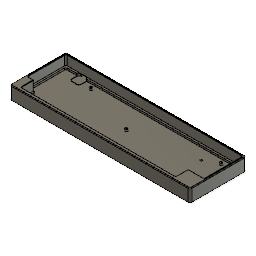
ttocyobitna (Autodesk Fusion 360 design; units mm, degrees)
Autodesk Fusion 360 part; units mm, degrees
sketch "Sketch1" plane through (0, 0, 0) normal (0, 1, 0) x (1, 0, 0)
  line L0 (0, 0) -> (274.2, 0)
  line L1 (274.2, 0) -> (274.2, -85.7)
  line L2 (274.2, -85.7) -> (0, -85.7)
  line L3 (0, -85.7) -> (0, 0)
  dimension "d1" = 274.2
  dimension "d2" = 85.7
  constraint horizontal L0
  constraint vertical L1
  constraint horizontal L2
  constraint vertical L3
  constraint coincident L0.start L3.end
  measures "d1" distance of L0.start L0.end
  measures "d2" distance of L0.start L2.end
extrude "Extrude1" add sketch "Sketch1" along normal blind 20.5
sketch "Sketch2" plane through (0, 20.5, 0) normal (0, 1, 0) x (-1, 0, 0)
  line L0 (0, 85.7) -> (-274.2, 85.7)
  line L1 (-274.2, 85.7) -> (-274.2, 0)
  line L2 (-274.2, 0) -> (0, 0)
  line L3 (0, 0) -> (0, 85.7)
  line L4 (-5, 3) -> (-269.2, 3)
  line L5 (-271.2, 5) -> (-271.2, 78.7)
  line L6 (-269.2, 80.7) -> (-5, 80.7)
  line L7 (-3, 78.7) -> (-3, 5)
  arc A0 (-5, 3) -> (-3, 5) centre (-5, 5) ccw
  arc A1 (-3, 78.7) -> (-5, 80.7) centre (-5, 78.7) ccw
  arc A2 (-269.2, 80.7) -> (-271.2, 78.7) centre (-269.2, 78.7) ccw
  arc A3 (-271.2, 5) -> (-269.2, 3) centre (-269.2, 5) ccw
  dimension "d5" = 3
  dimension "d6" = 5
  dimension "d7" = 3
  dimension "d8" = 3
  dimension "d9" = 2
  constraint horizontal L4
  constraint vertical L5
  constraint horizontal L6
  constraint vertical L7
  constraint tangent L4 A0
  constraint tangent L7 A0
  constraint tangent L6 A1
  constraint tangent L7 A1
  constraint equal A0 A1
  constraint tangent L5 A2
  constraint tangent L6 A2
  constraint equal A0 A2
  constraint tangent L4 A3
  constraint tangent L5 A3
  constraint equal A0 A3
  measures "d5" distance of L1 L5
  measures "d6" distance of L0 L6
  measures "d7" distance of L2 L4
  measures "d8" distance of L3 L7
  measures "d9" radius of A0
extrude "Extrude2" cut sketch "Sketch2" against normal blind 17.23 contours L4 L5 L6 L7 A0 A1 A2 A3
sketch "Sketch3" plane through (0, 3.27, 0) normal (0, 1, 0) x (-1, 0, 0)
  arc A0 (-269.2, 80.7) -> (-271.2, 78.7) centre (-269.2, 78.7) ccw
  line L0 (-271.2, 78.7) -> (-271.2, 5)
  arc A1 (-271.2, 5) -> (-269.2, 3) centre (-269.2, 5) ccw
  line L1 (-269.2, 3) -> (-5, 3)
  arc A2 (-5, 3) -> (-3, 5) centre (-5, 5) ccw
  line L2 (-3, 5) -> (-3, 78.7)
  arc A3 (-3, 78.7) -> (-5, 80.7) centre (-5, 78.7) ccw
  line L3 (-5, 80.7) -> (-269.2, 80.7)
  circle A4 centre (-51.375, 13.275) radius 2
  circle A5 centre (-36.275, 70.425) radius 2
  circle A6 centre (-132.3375, 40.775) radius 2
  circle A7 centre (-223.775, 70.425) radius 2
  circle A8 centre (-249.0188, 13.275) radius 2
  circle A9 centre (-228.275, 22.8) radius 1.5875
  line L4 (-7.75, 5.75) -> (-266.45, 5.75)
  line L5 (-268.45, 7.75) -> (-268.45, 75.95)
  line L6 (-266.45, 77.95) -> (-7.75, 77.95)
  line L7 (-5.75, 75.95) -> (-5.75, 7.75)
  arc A10 (-7.75, 5.75) -> (-5.75, 7.75) centre (-7.75, 7.75) ccw
  arc A11 (-5.75, 75.95) -> (-7.75, 77.95) centre (-7.75, 75.95) ccw
  arc A12 (-268.45, 7.75) -> (-266.45, 5.75) centre (-266.45, 7.75) ccw
  arc A13 (-266.45, 77.95) -> (-268.45, 75.95) centre (-266.45, 75.95) ccw
  line L8 (-22.9438, 3) -> (-36.9438, 3)
  line L9 (-36.9438, 3) -> (-36.9438, 17)
  line L10 (-36.9438, 17) -> (-22.9438, 17)
  line L11 (-22.9438, 17) -> (-22.9438, 3)
  point P0 (-13.275, 13.275)
  point P1 (-29.9438, 13.275)
  dimension "d12" = 10.275
  dimension "d13" = 10.275
  dimension "d14" = 4
  dimension "d15" = 38.1
  dimension "d16" = 4
  dimension "d17" = 57.15
  dimension "d18" = 23
  dimension "d19" = 4
  dimension "d20" = 4
  dimension "d21" = 4
  dimension "d22" = 119.0625
  dimension "d23" = 27.5
  dimension "d24" = 235.7438
  dimension "d25" = 210.5
  dimension "d26" = 57.15
  dimension "d27" = 3.175
  dimension "d28" = 215
  dimension "d29" = 9.525
  dimension "d30" = 2.75
  dimension "d31" = 2.75
  dimension "d32" = 2.75
  dimension "d33" = 2.75
  dimension "d34" = 2
  dimension "d41" = 16.6687
  dimension "d43" = 14
  dimension "d44" = 14
  dimension "d45" = 7
  constraint horizontal L4
  constraint vertical L5
  constraint horizontal L6
  constraint vertical L7
  constraint tangent L4 A10
  constraint tangent L7 A10
  constraint tangent L6 A11
  constraint tangent L7 A11
  constraint equal A10 A11
  constraint tangent L4 A12
  constraint tangent L5 A12
  constraint equal A10 A12
  constraint tangent L5 A13
  constraint tangent L6 A13
  constraint equal A10 A13
  constraint horizontal L8
  constraint vertical L9
  constraint horizontal L10
  constraint vertical L11
  constraint coincident L1 L8.start
  measures "d12" distance of L1 P0
  measures "d13" distance of L2 P0
  measures "d14" diameter of A4
  measures "d15" distance of P0 A4.centre
  measures "d16" diameter of A5
  measures "d17" vertical distance of P0 A5.centre
  measures "d18" horizontal distance of P0 A5.centre
  measures "d19" diameter of A6
  measures "d20" diameter of A7
  measures "d21" diameter of A8
  measures "d22" horizontal distance of P0 A6.centre
  measures "d23" vertical distance of P0 A6.centre
  measures "d24" distance of P0 A8.centre
  measures "d25" horizontal distance of P0 A7.centre
  measures "d26" vertical distance of P0 A7.centre
  measures "d27" diameter of A9
  measures "d28" horizontal distance of P0 A9.centre
  measures "d29" vertical distance of P0 A9.centre
  measures "d30" distance of L1 L4
  measures "d31" distance of L0 L5
  measures "d32" distance of L3 L6
  measures "d33" distance of L2 L7
  measures "d34" radius of A10
  measures "d41" distance of P0 P1
  measures "d43" distance of L8.start L8.end
  measures "d44" distance of L8.start L10.end
  measures "d45" distance of P1 L11
extrude "Extrude5" cut sketch "Sketch3" against normal blind 0.52 contours L1 L4 L8 L9 L11 | L4 L9 L10 L11
extrude "Extrude3" add sketch "Sketch3" along normal blind 2.73 contours A0 L0 A1 L1 A2 L2 A3 L3 L4 L5 L6 L7 A10 A11 A12 A13 L9 L11 | L1 L4 L8 L9 L11 | A4 | A5 | A6 | A7 | A8
extrude "Extrude4" cut sketch "Sketch3" against normal blind 3.27 contours A9
sketch "Sketch4" plane through (0, 0, 0) normal (0, 0, -1) x (-1, 0, 0)
  line L0 (-274.2, 0) -> (0, 0)
  line L1 (0, 0) -> (0, 20.5)
  line L2 (0, 20.5) -> (-274.2, 20.5)
  line L3 (-274.2, 20.5) -> (-274.2, 0)
  line L4 (-33.4438, 6.25) -> (-26.4438, 6.25)
  line L5 (-25.4438, 5.25) -> (-25.4438, 3.75)
  line L6 (-26.4438, 2.75) -> (-33.4437, 2.75)
  line L7 (-34.4438, 3.75) -> (-34.4437, 5.25)
  arc A0 (-33.4438, 6.25) -> (-34.4438, 5.25) centre (-33.4438, 5.25) ccw
  arc A1 (-34.4438, 3.75) -> (-33.4438, 2.75) centre (-33.4438, 3.75) ccw
  arc A2 (-26.4438, 2.75) -> (-25.4438, 3.75) centre (-26.4438, 3.75) ccw
  arc A3 (-25.4438, 5.25) -> (-26.4438, 6.25) centre (-26.4438, 5.25) ccw
  point P0 (-55.875, 6.25)
  point P1 (-55.875, 2.75)
  point P2 (-51.375, 3.27)
  point P3 (-34.4438, 6.25)
  point P4 (-25.4438, 6.25)
  point P5 (-34.4438, 2.75)
  point P6 (-29.9438, 3.27)
  dimension "d53" = 9
  dimension "d54" = 3.5
  dimension "d55" = 4.5
  dimension "d56" = 2.98
  dimension "d57" = 1
  constraint horizontal L4
  constraint vertical L5
  constraint horizontal L6
  constraint vertical L7
  constraint coincident P3 L4
  constraint coincident P3 L7
  constraint tangent L4 A0
  constraint tangent L7 A0
  constraint coincident P5 L6
  constraint coincident P5 L7
  constraint tangent L6 A1
  constraint tangent L7 A1
  constraint equal A0 A1
  constraint tangent L5 A2
  constraint tangent L6 A2
  constraint equal A0 A2
  constraint coincident P4 L4
  constraint coincident P4 L5
  constraint tangent L4 A3
  constraint tangent L5 A3
  constraint equal A0 A3
  measures "d53" distance of P3 P4
  measures "d54" distance of P3 P5
  measures "d55" distance of L5 P6
  measures "d56" distance of L4 P6
  measures "d57" radius of A0
extrude "Extrude6" cut sketch "Sketch4" against normal blind 3 contours L4 L5 L6 L7 A0 A1 A2 A3
extrude "Extrude7" cut sketch "Sketch3" along normal blind 2.73 contours L1 L4 L8 L9 L11
fillet "Fillet1" radius 3.175 1 edges at (22.9438, 4.375, 3)
fillet "Fillet2" radius 3.175 1 edges at (36.9438, 4.375, 3)
fillet "Fillet3" radius 3.175 2 edges at (36.9438, 3.01, 17) (22.9438, 3.01, 17)
sketch "Sketch5" plane through (0, 20.5, 0) normal (0, 1, 0) x (-1, 0, 0)
  line L0 (-271.2, 5) -> (-271.2, 78.7)
  arc A0 (-269.2, 80.7) -> (-271.2, 78.7) centre (-269.2, 78.7) ccw
  line L1 (-269.2, 80.7) -> (-5, 80.7)
  arc A1 (-3, 78.7) -> (-5, 80.7) centre (-5, 78.7) ccw
  line L2 (-3, 78.7) -> (-3, 5)
  arc A2 (-5, 3) -> (-3, 5) centre (-5, 5) ccw
  line L3 (-5, 3) -> (-269.2, 3)
  arc A3 (-271.2, 5) -> (-269.2, 3) centre (-269.2, 5) ccw
  line L4 (0, 85.7) -> (-274.2, 85.7)
  line L5 (-274.2, 85.7) -> (-274.2, 0)
  line L6 (-274.2, 0) -> (0, 0)
  line L7 (0, 0) -> (0, 85.7)
  line L8 (-12.525, 80.7) -> (-3, 80.7)
  line L9 (-3, 80.7) -> (-3, 61.65)
  line L10 (-3, 61.65) -> (-12.525, 61.65)
  line L11 (-12.525, 61.65) -> (-12.525, 80.7)
  line L12 (-271.2, 61.65) -> (-247.3875, 61.65)
  line L13 (-247.3875, 61.65) -> (-247.3875, 80.7)
  line L14 (-247.3875, 80.7) -> (-271.2, 80.7)
  line L15 (-271.2, 80.7) -> (-271.2, 61.65)
  dimension "d65" = 9.525
  dimension "d66" = 19.05
  dimension "d67" = 19.05
  dimension "d68" = 23.8125
  constraint horizontal L8
  constraint vertical L9
  constraint horizontal L10
  constraint vertical L11
  constraint coincident L2 L9.end
  constraint horizontal L12
  constraint vertical L13
  constraint horizontal L14
  constraint vertical L15
  constraint coincident L1 L13.end
  constraint coincident L0 L12.start
  measures "d65" distance of L9.end L10.end
  measures "d66" distance of L8.start L10.end
  measures "d67" distance of L12.end L13.end
  measures "d68" distance of L12.start L12.end
extrude "Extrude8" add sketch "Sketch5" against normal blind 20.5 contours L0 A0 L1 L12 L13 L14 L15 | L1 A1 L2 L8 L9 L10 L11
fillet "Fillet4" radius 2 2 edges at (3, 13.25, 61.65) (12.525, 13.25, 80.7)
fillet "Fillet5" radius 2 2 edges at (271.2, 13.25, 61.65) (247.3875, 13.25, 80.7)
fillet "Fillet6" radius 0.5 1 edges at (247.3875, 11.885, 61.65)
fillet "Fillet7" radius 0.5 1 edges at (12.525, 11.885, 61.65)
sketch "Sketch6" plane through (0, 3.27, 0) normal (0, 1, 0) x (-1, 0, 0)
  line L0 (-12.525, 62.15) -> (-12.525, 77.95)
  line L1 (-12.525, 77.95) -> (-247.3875, 77.95)
  line L2 (-247.3875, 77.95) -> (-247.3875, 62.15)
  arc A0 (-247.8875, 61.65) -> (-247.3875, 62.15) centre (-247.8875, 62.15) ccw
  line L3 (-247.8875, 61.65) -> (-268.45, 61.65)
  line L4 (-268.45, 61.65) -> (-268.45, 7.75)
  arc A1 (-268.45, 7.75) -> (-266.45, 5.75) centre (-266.45, 7.75) ccw
  line L5 (-266.45, 5.75) -> (-36.9152, 5.75)
  arc A2 (-36.9438, 6.175) -> (-36.9152, 5.75) centre (-33.7688, 6.175) ccw
  line L6 (-36.9438, 6.175) -> (-36.9438, 13.825)
  arc A3 (-33.7688, 17) -> (-36.9438, 13.825) centre (-33.7688, 13.825) ccw
  line L7 (-33.7688, 17) -> (-26.1188, 17)
  arc A4 (-22.9438, 13.825) -> (-26.1188, 17) centre (-26.1188, 13.825) ccw
  line L8 (-22.9438, 13.825) -> (-22.9438, 6.175)
  arc A5 (-22.9723, 5.75) -> (-22.9438, 6.175) centre (-26.1188, 6.175) ccw
  line L9 (-22.9723, 5.75) -> (-7.75, 5.75)
  arc A6 (-7.75, 5.75) -> (-5.75, 7.75) centre (-7.75, 7.75) ccw
  line L10 (-5.75, 7.75) -> (-5.75, 61.65)
  line L11 (-5.75, 61.65) -> (-12.025, 61.65)
  arc A7 (-12.525, 62.15) -> (-12.025, 61.65) centre (-12.025, 62.15) ccw
  circle A8 centre (-228.275, 22.8) radius 1.5875
  circle A9 centre (-249.0188, 13.275) radius 2
  circle A10 centre (-51.375, 13.275) radius 2
  circle A11 centre (-36.275, 70.425) radius 2
  circle A12 centre (-223.775, 70.425) radius 2
  circle A13 centre (-132.3375, 40.775) radius 2
  line L12 (-15.275, 77.95) -> (-12.525, 77.95)
  line L13 (-12.525, 77.95) -> (-12.525, 58.9)
  line L14 (-12.525, 58.9) -> (-12.525, 58.9)
  line L15 (-15.275, 61.65) -> (-15.275, 77.95)
  line L16 (-12.525, 58.9) -> (-5.75, 58.9)
  line L17 (-5.75, 58.9) -> (-5.75, 61.65)
  line L18 (-5.75, 61.65) -> (-12.525, 61.65)
  line L19 (-12.525, 61.65) -> (-12.525, 58.9)
  arc A14 (-15.275, 61.65) -> (-12.525, 58.9) centre (-12.525, 61.65) ccw
  dimension "d75" = 2.75
  dimension "d77" = 2.75
  constraint horizontal L12
  constraint vertical L13
  constraint vertical L15
  constraint coincident L1 L12.start
  constraint horizontal L16
  constraint vertical L17
  constraint horizontal L18
  constraint vertical L19
  constraint coincident L10.end L11.start
  constraint tangent L15 A14
  measures "d75" distance of L13 L15
  measures "d77" radius of A14
extrude "Extrude9" add sketch "Sketch6" along normal blind 2.73 contours L0 L1 L12 L13 L15 L19 A14 | A7 L13 L18 | L10 L11 L13 L16 L17 L18 L19
sketch "Sketch7" plane through (0, 3.27, 0) normal (0, 1, 0) x (-1, 0, 0)
  line L0 (-15.275, 61.65) -> (-15.275, 77.95)
  line L1 (-15.275, 77.95) -> (-247.3875, 77.95)
  line L2 (-247.3875, 77.95) -> (-247.3875, 62.15)
  arc A0 (-247.8875, 61.65) -> (-247.3875, 62.15) centre (-247.8875, 62.15) ccw
  line L3 (-247.8875, 61.65) -> (-268.45, 61.65)
  line L4 (-268.45, 61.65) -> (-268.45, 7.75)
  arc A1 (-268.45, 7.75) -> (-266.45, 5.75) centre (-266.45, 7.75) ccw
  line L5 (-266.45, 5.75) -> (-36.9152, 5.75)
  arc A2 (-36.9438, 6.175) -> (-36.9152, 5.75) centre (-33.7688, 6.175) ccw
  line L6 (-36.9438, 6.175) -> (-36.9438, 13.825)
  arc A3 (-33.7688, 17) -> (-36.9438, 13.825) centre (-33.7688, 13.825) ccw
  line L7 (-33.7688, 17) -> (-26.1188, 17)
  arc A4 (-22.9438, 13.825) -> (-26.1188, 17) centre (-26.1188, 13.825) ccw
  line L8 (-22.9438, 13.825) -> (-22.9438, 6.175)
  arc A5 (-22.9723, 5.75) -> (-22.9438, 6.175) centre (-26.1188, 6.175) ccw
  line L9 (-22.9723, 5.75) -> (-7.75, 5.75)
  arc A6 (-7.75, 5.75) -> (-5.75, 7.75) centre (-7.75, 7.75) ccw
  line L10 (-5.75, 7.75) -> (-5.75, 58.9)
  line L11 (-5.75, 58.9) -> (-12.525, 58.9)
  arc A7 (-15.275, 61.65) -> (-12.525, 58.9) centre (-12.525, 61.65) ccw
  circle A8 centre (-228.275, 22.8) radius 1.5875
  circle A9 centre (-249.0188, 13.275) radius 2
  circle A10 centre (-51.375, 13.275) radius 2
  circle A11 centre (-36.275, 70.425) radius 2
  circle A12 centre (-223.775, 70.425) radius 2
  circle A13 centre (-132.3375, 40.775) radius 2
  line L12 (-244.6375, 77.95) -> (-247.3875, 77.95)
  line L13 (-247.3875, 77.95) -> (-247.3875, 58.9)
  line L14 (-247.3875, 58.9) -> (-247.3875, 58.9)
  line L15 (-244.6375, 61.65) -> (-244.6375, 77.95)
  line L16 (-247.3875, 58.9) -> (-268.45, 58.9)
  line L17 (-268.45, 58.9) -> (-268.45, 61.65)
  line L18 (-268.45, 61.65) -> (-247.3875, 61.65)
  line L19 (-247.3875, 61.65) -> (-247.3875, 58.9)
  arc A14 (-247.3875, 58.9) -> (-244.6375, 61.65) centre (-247.3875, 61.65) ccw
  point P0 (-244.6375, 58.9)
  dimension "d80" = 2.75
  dimension "d82" = 2.75
  constraint horizontal L12
  constraint vertical L13
  constraint vertical L15
  constraint coincident L1 L12.start
  constraint horizontal L16
  constraint vertical L17
  constraint horizontal L18
  constraint vertical L19
  constraint coincident L3.end L4.start
  constraint coincident P0 L14
  constraint coincident P0 L15
  constraint tangent L15 A14
  measures "d80" distance of L13.end P0
  measures "d82" radius of A14
extrude "Extrude10" add sketch "Sketch7" along normal blind 2.73 contours L1 L2 L12 L13 L15 L19 A14 | A0 L13 L18 | L3 L4 L13 L16 L17 L18 L19
sketch "Sketch8" plane through (0, 6, 0) normal (0, 1, 0) x (-1, 0, 0)
  circle A0 centre (-51.375, 13.275) radius 2
  circle A1 centre (-51.375, 13.275) radius 2
  constraint concentric A0 A1
sketch "Sketch9" plane through (0, 6, 0) normal (0, 1, 0) x (-1, 0, 0)
  circle A0 centre (-132.3375, 40.775) radius 2
  circle A1 centre (-132.3375, 40.775) radius 2
  constraint concentric A0 A1
sketch "Sketch10" plane through (0, 6, 0) normal (0, 1, 0) x (-1, 0, 0)
  circle A0 centre (-249.0188, 13.275) radius 2
  circle A1 centre (-249.0188, 13.275) radius 2
  constraint concentric A0 A1
sketch "Sketch11" plane through (0, 6, 0) normal (0, 1, 0) x (-1, 0, 0)
  circle A0 centre (-223.775, 70.425) radius 2
  circle A1 centre (-223.775, 70.425) radius 2
  constraint concentric A0 A1
sketch "Sketch12" plane through (0, 6, 0) normal (0, 1, 0) x (-1, 0, 0)
  circle A0 centre (-36.275, 70.425) radius 2
  circle A1 centre (-36.275, 70.425) radius 2
  constraint concentric A0 A1
hole "Hole1" at (51.375, 6, 13.275) direction (0, -1, 0) diameter 1.623 depth 4 tip angle 118
thread "Thread1" "ISO Metric profile 2.0 M2x0.4 6H"
hole "Hole2" at (132.3375, 6, 40.775) direction (0, -1, 0) diameter 1.623 depth 4 tip angle 118
thread "Thread2" "ISO Metric profile 2.0 M2x0.4 6H"
hole "Hole3" at (249.0188, 6, 13.275) direction (0, -1, 0) diameter 1.623 depth 4 tip angle 118
thread "Thread3" "ISO Metric profile 2.0 M2x0.4 6H"
hole "Hole4" at (223.775, 6, 70.425) direction (0, -1, 0) diameter 1.623 depth 4 tip angle 118
thread "Thread4" "ISO Metric profile 2.0 M2x0.4 6H"
hole "Hole5" at (36.275, 6, 70.425) direction (0, -1, 0) diameter 1.623 depth 4 tip angle 118
thread "Thread5" "ISO Metric profile 2.0 M2x0.4 6H"
sketch "Sketch13" plane through (0, 6, 0) normal (0, 1, 0) x (-1, 0, 0)
  arc A0 (-269.2, 61.65) -> (-271.2, 59.65) centre (-269.2, 59.65) ccw
  line L0 (-271.2, 59.65) -> (-271.2, 5)
  arc A1 (-271.2, 5) -> (-269.2, 3) centre (-269.2, 5) ccw
  line L1 (-269.2, 3) -> (-34.1052, 3)
  line L2 (-34.1052, 3) -> (-34.1052, 3.0179)
  arc A2 (-36.9152, 5.75) -> (-34.1052, 3.0179) centre (-33.7688, 6.175) ccw
  line L3 (-36.9152, 5.75) -> (-266.45, 5.75)
  arc A3 (-268.45, 7.75) -> (-266.45, 5.75) centre (-266.45, 7.75) ccw
  line L4 (-268.45, 7.75) -> (-268.45, 58.9)
  line L5 (-268.45, 58.9) -> (-247.3875, 58.9)
  arc A4 (-247.3875, 58.9) -> (-244.6375, 61.65) centre (-247.3875, 61.65) ccw
  line L6 (-244.6375, 61.65) -> (-244.6375, 77.95)
  line L7 (-244.6375, 77.95) -> (-15.275, 77.95)
  line L8 (-15.275, 77.95) -> (-15.275, 61.65)
  arc A5 (-15.275, 61.65) -> (-12.525, 58.9) centre (-12.525, 61.65) ccw
  line L9 (-12.525, 58.9) -> (-5.75, 58.9)
  line L10 (-5.75, 58.9) -> (-5.75, 7.75)
  arc A6 (-7.75, 5.75) -> (-5.75, 7.75) centre (-7.75, 7.75) ccw
  line L11 (-7.75, 5.75) -> (-22.9723, 5.75)
  arc A7 (-25.7823, 3.0179) -> (-22.9723, 5.75) centre (-26.1188, 6.175) ccw
  line L12 (-25.7823, 3.0179) -> (-25.7823, 3)
  line L13 (-25.7823, 3) -> (-5, 3)
  arc A8 (-5, 3) -> (-3, 5) centre (-5, 5) ccw
  line L14 (-3, 5) -> (-3, 59.65)
  arc A9 (-3, 59.65) -> (-5, 61.65) centre (-5, 59.65) ccw
  line L15 (-5, 61.65) -> (-12.025, 61.65)
  arc A10 (-12.525, 62.15) -> (-12.025, 61.65) centre (-12.025, 62.15) ccw
  line L16 (-12.525, 62.15) -> (-12.525, 78.7)
  arc A11 (-12.525, 78.7) -> (-14.525, 80.7) centre (-14.525, 78.7) ccw
  line L17 (-14.525, 80.7) -> (-245.3875, 80.7)
  arc A12 (-245.3875, 80.7) -> (-247.3875, 78.7) centre (-245.3875, 78.7) ccw
  line L18 (-247.3875, 78.7) -> (-247.3875, 62.15)
  arc A13 (-247.8875, 61.65) -> (-247.3875, 62.15) centre (-247.8875, 62.15) ccw
  line L19 (-247.8875, 61.65) -> (-269.2, 61.65)
  line L20 (-5.75, 58.9) -> (-5.75, 61.65)
  line L21 (-11.6734, 61.65) -> (-15.275, 61.65)
  constraint coincident L9.end L10.start
  constraint perpendicular L15 L20
  constraint coincident L15 L20.end
  constraint coincident L15 L21.start
  constraint perpendicular L8 L21
extrude "Extrude11" cut sketch "Sketch13" against normal blind 2.73 contours A5 L9 L15 L20 L21
fillet "Fillet8" radius 2 1 edges at (5.75, 4.635, 61.65)
fillet "Fillet9" radius 2 1 edges at (15.275, 4.635, 61.65)
sketch "Sketch14" plane through (0, 6, 0) normal (0, 1, 0) x (-1, 0, 0)
  arc A0 (-15.275, 63.65) -> (-13.275, 61.65) centre (-13.275, 63.65) ccw
  line L0 (-13.275, 61.65) -> (-12.025, 61.65)
  arc A1 (-12.525, 62.15) -> (-12.025, 61.65) centre (-12.025, 62.15) ccw
  line L1 (-12.525, 62.15) -> (-12.525, 78.7)
  arc A2 (-12.525, 78.7) -> (-14.525, 80.7) centre (-14.525, 78.7) ccw
  line L2 (-14.525, 80.7) -> (-245.3875, 80.7)
  arc A3 (-245.3875, 80.7) -> (-247.3875, 78.7) centre (-245.3875, 78.7) ccw
  line L3 (-247.3875, 78.7) -> (-247.3875, 62.15)
  arc A4 (-247.8875, 61.65) -> (-247.3875, 62.15) centre (-247.8875, 62.15) ccw
  line L4 (-247.8875, 61.65) -> (-269.2, 61.65)
  arc A5 (-269.2, 61.65) -> (-271.2, 59.65) centre (-269.2, 59.65) ccw
  line L5 (-271.2, 59.65) -> (-271.2, 5)
  arc A6 (-271.2, 5) -> (-269.2, 3) centre (-269.2, 5) ccw
  line L6 (-269.2, 3) -> (-34.1052, 3)
  line L7 (-34.1052, 3) -> (-34.1052, 3.0179)
  arc A7 (-36.9152, 5.75) -> (-34.1052, 3.0179) centre (-33.7688, 6.175) ccw
  line L8 (-36.9152, 5.75) -> (-266.45, 5.75)
  arc A8 (-268.45, 7.75) -> (-266.45, 5.75) centre (-266.45, 7.75) ccw
  line L9 (-268.45, 7.75) -> (-268.45, 58.9)
  line L10 (-268.45, 58.9) -> (-247.3875, 58.9)
  arc A9 (-247.3875, 58.9) -> (-244.6375, 61.65) centre (-247.3875, 61.65) ccw
  line L11 (-244.6375, 61.65) -> (-244.6375, 77.95)
  line L12 (-244.6375, 77.95) -> (-15.275, 77.95)
  line L13 (-15.275, 77.95) -> (-15.275, 63.65)
  line L14 (-84.6015, 77.95) -> (-187.0892, 77.95)
  line L15 (-187.0892, 77.95) -> (-187.0892, 80.7)
  line L16 (-187.0892, 80.7) -> (-84.6015, 80.7)
  line L17 (-84.6015, 80.7) -> (-84.6015, 77.95)
  constraint horizontal L14
  constraint vertical L15
  constraint horizontal L16
  constraint vertical L17
  constraint coincident L2 L15.end
  constraint coincident L12 L14.start
extrude "Extrude12" cut sketch "Sketch14" against normal blind 2.73 contours L2 L12 L14 L15 L16 L17
fillet "Fillet10" radius 2 1 edges at (84.6015, 4.635, 77.95)
fillet "Fillet11" radius 2 1 edges at (187.0892, 4.635, 77.95)
fillet "Fillet12" radius 2 1 edges at (84.6015, 4.635, 80.7)
fillet "Fillet13" radius 2 1 edges at (187.0892, 4.635, 80.7)
chamfer "Chamfer1" distance 0.5 angle 45 16 edges at (271.2, 20.5, 32.325) (270.6142, 20.5, 61.0642) (258.5438, 20.5, 61.65) (247.5339, 20.5, 61.7964) (247.3875, 20.5, 70.425) (246.8017, 20.5, 80.1142) (129.9562, 20.5, 80.7) (13.1108, 20.5, 80.1142) (12.525, 20.5, 70.425) (12.3786, 20.5, 61.7964) (8.5125, 20.5, 61.65) (3.5858, 20.5, 61.0642) (3, 20.5, 32.325) (3.5858, 20.5, 3.5858) (137.1, 20.5, 3) (270.6142, 20.5, 3.5858)
fillet "Fillet14" radius 3 3 edges at (0, 10.25, 85.7) (0, 10.25, 0) (274.2, 10.25, 85.7)
fillet "Fillet15" radius 3 1 edges at (274.2, 10.25, 0)
chamfer "Chamfer2" distance 1 angle 45 8 edges at (273.3213, 20.5, 84.8213) (274.2, 20.5, 42.85) (273.3213, 20.5, 0.8787) (137.1, 20.5, 0) (0.8787, 20.5, 0.8787) (0, 20.5, 42.85) (0.8787, 20.5, 84.8213) (137.1, 20.5, 85.7)
sketch "Sketch15" plane through (0, 20.5, 0) normal (0, 1, 0) x (-1, 0, 0)
  line L0 (-271.7, 5) -> (-271.7, 59.65)
  arc A0 (-269.2, 62.15) -> (-271.7, 59.65) centre (-269.2, 59.65) ccw
  line L1 (-269.2, 62.15) -> (-247.8875, 62.15)
  line L2 (-247.8875, 62.15) -> (-247.8875, 78.7)
  arc A1 (-245.3875, 81.2) -> (-247.8875, 78.7) centre (-245.3875, 78.7) ccw
  line L3 (-245.3875, 81.2) -> (-14.525, 81.2)
  arc A2 (-12.025, 78.7) -> (-14.525, 81.2) centre (-14.525, 78.7) ccw
  line L4 (-12.025, 78.7) -> (-12.025, 62.15)
  line L5 (-12.025, 62.15) -> (-5, 62.15)
  arc A3 (-2.5, 59.65) -> (-5, 62.15) centre (-5, 59.65) ccw
  line L6 (-2.5, 59.65) -> (-2.5, 5)
  arc A4 (-5, 2.5) -> (-2.5, 5) centre (-5, 5) ccw
  line L7 (-5, 2.5) -> (-269.2, 2.5)
  arc A5 (-271.7, 5) -> (-269.2, 2.5) centre (-269.2, 5) ccw
  arc A6 (-271.2, 84.7) -> (-273.2, 82.7) centre (-271.2, 82.7) ccw
  line L8 (-273.2, 82.7) -> (-273.2, 3)
  arc A7 (-273.2, 3) -> (-271.2, 1) centre (-271.2, 3) ccw
  line L9 (-271.2, 1) -> (-3, 1)
  arc A8 (-3, 1) -> (-1, 3) centre (-3, 3) ccw
  line L10 (-1, 3) -> (-1, 82.7)
  arc A9 (-1, 82.7) -> (-3, 84.7) centre (-3, 82.7) ccw
  line L11 (-3, 84.7) -> (-271.2, 84.7)
  line L12 (0, 7) -> (-3, 7)
  line L13 (-3, 7) -> (-3, 9)
  line L14 (-3, 9) -> (0, 9)
  line L15 (0, 9) -> (0, 7)
  line L16 (0, 3) -> (0, 82.7)
  line L17 (-3, 59.65) -> (-3, 5)
  line L18 (-3, 5) -> (-2.5, 5)
  line L19 (-3, 9) -> (0, 9)
  line L20 (0, 9) -> (0, 11)
  line L21 (0, 11) -> (-3, 11)
  line L22 (-3, 11) -> (-3, 9)
  line L23 (-3, 11) -> (0, 11)
  line L24 (0, 11) -> (0, 13)
  line L25 (0, 13) -> (-3, 13)
  line L26 (-3, 13) -> (-3, 11)
  line L27 (-3, 13) -> (0, 13)
  line L28 (0, 13) -> (0, 15)
  line L29 (0, 15) -> (-3, 15)
  line L30 (-3, 15) -> (-3, 13)
  line L31 (-3, 15) -> (0, 15)
  line L32 (0, 15) -> (0, 17)
  line L33 (0, 17) -> (-3, 17)
  line L34 (-3, 17) -> (-3, 15)
  line L35 (-3, 17) -> (0, 17)
  line L36 (0, 17) -> (0, 19)
  line L37 (0, 19) -> (-3, 19)
  line L38 (-3, 19) -> (-3, 17)
  line L39 (-3, 19) -> (0, 19)
  line L40 (0, 19) -> (0, 21)
  line L41 (0, 21) -> (-3, 21)
  line L42 (-3, 21) -> (-3, 19)
  line L43 (-3, 21) -> (0, 21)
  line L44 (0, 21) -> (0, 23)
  line L45 (0, 23) -> (-3, 23)
  line L46 (-3, 23) -> (-3, 21)
  line L47 (-3, 23) -> (0, 23)
  line L48 (0, 23) -> (0, 25)
  line L49 (0, 25) -> (-3, 25)
  line L50 (-3, 25) -> (-3, 23)
  line L51 (-3, 25) -> (0, 25)
  line L52 (0, 25) -> (0, 27)
  line L53 (0, 27) -> (-3, 27)
  line L54 (-3, 27) -> (-3, 25)
  line L55 (-3, 5) -> (0, 5)
  line L56 (0, 5) -> (0, 7)
  line L57 (0, 7) -> (-3, 7)
  line L58 (-3, 7) -> (-3, 5)
  line L59 (-3, 27) -> (0, 27)
  line L60 (0, 27) -> (0, 29)
  line L61 (0, 29) -> (-3, 29)
  line L62 (-3, 29) -> (-3, 27)
  line L63 (-3, 29) -> (0, 29)
  line L64 (0, 29) -> (0, 31)
  line L65 (0, 31) -> (-3, 31)
  line L66 (-3, 31) -> (-3, 29)
  line L67 (-3, 31) -> (0, 31)
  line L68 (0, 31) -> (0, 33)
  line L69 (0, 33) -> (-3, 33)
  line L70 (-3, 33) -> (-3, 31)
  line L71 (-3, 33) -> (0, 33)
  line L72 (0, 33) -> (0, 35)
  line L73 (0, 35) -> (-3, 35)
  line L74 (-3, 35) -> (-3, 33)
  line L75 (-3, 35) -> (0, 35)
  line L76 (0, 35) -> (0, 37)
  line L77 (0, 37) -> (-3, 37)
  line L78 (-3, 37) -> (-3, 35)
  line L79 (-3, 37) -> (0, 37)
  line L80 (0, 37) -> (0, 39)
  line L81 (0, 39) -> (-3, 39)
  line L82 (-3, 39) -> (-3, 37)
  line L83 (-3, 39) -> (0, 39)
  line L84 (0, 39) -> (0, 41)
  line L85 (0, 41) -> (-3, 41)
  line L86 (-3, 41) -> (-3, 39)
  dimension "d114" = 2
  dimension "d115" = 2
  dimension "d116" = 2
  dimension "d117" = 2
  dimension "d118" = 2
  dimension "d119" = 2
  dimension "d120" = 2
  dimension "d121" = 2
  dimension "d122" = 2
  dimension "d123" = 2
  dimension "d124" = 2
  dimension "d142" = 2
  dimension "d143" = 2
  dimension "d144" = 2
  dimension "d145" = 2
  dimension "d146" = 2
  dimension "d147" = 2
  dimension "d148" = 2
  constraint horizontal L12
  constraint vertical L13
  constraint horizontal L14
  constraint vertical L15
  constraint coincident L13.end L17
  constraint coincident L12.start L16
  constraint horizontal L19
  constraint vertical L20
  constraint horizontal L21
  constraint vertical L22
  constraint coincident L16 L20.end
  constraint horizontal L23
  constraint vertical L24
  constraint horizontal L25
  constraint vertical L26
  constraint coincident L16 L24.end
  constraint horizontal L27
  constraint vertical L28
  constraint horizontal L29
  constraint vertical L30
  constraint coincident L16 L28.end
  constraint horizontal L31
  constraint vertical L32
  constraint horizontal L33
  constraint vertical L34
  constraint coincident L16 L32.end
  constraint horizontal L35
  constraint vertical L36
  constraint horizontal L37
  constraint vertical L38
  constraint coincident L16 L36.end
  constraint horizontal L39
  constraint vertical L40
  constraint horizontal L41
  constraint vertical L42
  constraint coincident L16 L40.end
  constraint horizontal L43
  constraint vertical L44
  constraint horizontal L45
  constraint vertical L46
  constraint coincident L16 L44.end
  constraint horizontal L47
  constraint vertical L48
  constraint horizontal L49
  constraint vertical L50
  constraint coincident L16 L48.end
  constraint horizontal L51
  constraint vertical L52
  constraint horizontal L53
  constraint vertical L54
  constraint coincident L16 L52.end
  constraint horizontal L55
  constraint vertical L56
  constraint horizontal L57
  constraint vertical L58
  constraint coincident L17.end L18.start
  constraint horizontal L59
  constraint vertical L60
  constraint horizontal L61
  constraint vertical L62
  constraint horizontal L63
  constraint vertical L64
  constraint horizontal L65
  constraint vertical L66
  constraint horizontal L67
  constraint vertical L68
  constraint horizontal L69
  constraint vertical L70
  constraint horizontal L71
  constraint vertical L72
  constraint horizontal L73
  constraint vertical L74
  constraint horizontal L75
  constraint vertical L76
  constraint horizontal L77
  constraint vertical L78
  constraint horizontal L79
  constraint vertical L80
  constraint horizontal L81
  constraint vertical L82
  constraint horizontal L83
  constraint vertical L84
  constraint horizontal L85
  constraint vertical L86
  measures "d114" distance of L12 L18
  measures "d115" distance of L12.start L14.end
  measures "d116" distance of L14.end L20.end
  measures "d117" distance of L20.end L24.end
  measures "d118" distance of L24.end L28.end
  measures "d119" distance of L28.end L32.end
  measures "d120" distance of L32.end L36.end
  measures "d121" distance of L36.end L40.end
  measures "d122" distance of L40.end L44.end
  measures "d123" distance of L44.end L48.end
  measures "d124" distance of L48.end L52.end
  measures "d142" distance of L53.end L61.end
  measures "d143" distance of L61.end L65.end
  measures "d144" distance of L65.end L69.end
  measures "d145" distance of L69.end L73.end
  measures "d146" distance of L73.end L77.end
  measures "d147" distance of L77.end L81.end
  measures "d148" distance of L81.end L85.end
extrude "Extrude13" cut sketch "Sketch15" against normal blind 1 contours L6 L14 L17 L19 L21 L22 L23 | L6 L10 L14 L19 L21 L23 | L10 L14 L16 L19 L20 L21 L23 | L6 L17 L25 L27 L29 L30 L31 | L6 L10 L25 L27 L29 L31 | L10 L16 L25 L27 L28 L29 L31 | L6 L17 L33 L35 L37 L38 L39 | L6 L10 L33 L35 L37 L39 | L10 L16 L33 L35 L36 L37 L39 | L6 L17 L41 L43 L45 L46 L47 | L6 L10 L41 L43 L45 L47 | L6 L10 L77 L79 L81 L83 | L6 L17 L77 L79 L81 L82 L83 | L10 L16 L41 L43 L44 L45 L47 | L10 L16 L77 L79 L80 L81 L83 | L6 L17 L49 L51 L53 L54 L59 | L6 L10 L49 L51 L53 L59 | L6 L10 L69 L71 L73 L75 | L6 L17 L69 L71 L73 L74 L75 | L10 L16 L49 L51 L52 L53 L59 | L10 L16 L69 L71 L72 L73 L75 | L6 L17 L61 L63 L65 L66 L67 | L6 L10 L61 L63 L65 L67 | L10 L16 L61 L63 L64 L65 L67
chamfer "Chamfer3" distance 1 angle 45 8 edges at (273.3213, 0, 0.8787) (274.2, 0, 42.85) (273.3213, 0, 84.8213) (137.1, 0, 85.7) (0.8787, 0, 84.8213) (0, 0, 42.85) (0.8787, 0, 0.8787) (137.1, 0, 0)
sketch "Sketch16" plane through (0, 0, 0) normal (0, -1, 0) x (1, 0, 0)
  circle A0 centre (228.275, 22.8) radius 1.5875
  arc A1 (271.2, 1) -> (273.2, 3) centre (271.2, 3) ccw
  line L0 (273.2, 3) -> (273.2, 82.7)
  arc A2 (273.2, 82.7) -> (271.2, 84.7) centre (271.2, 82.7) ccw
  line L1 (271.2, 84.7) -> (3, 84.7)
  arc A3 (3, 84.7) -> (1, 82.7) centre (3, 82.7) ccw
  line L2 (1, 82.7) -> (1, 3)
  arc A4 (1, 3) -> (3, 1) centre (3, 3) ccw
  line L3 (3, 1) -> (271.2, 1)
  circle A5 centre (13, 72.7) radius 9.775
  line L4 (271.2, 85.7) -> (3, 85.7)
  line L5 (0, 82.7) -> (0, 3)
  circle A6 centre (13, 13) radius 9.775
  line L6 (3, 0) -> (271.2, 0)
  circle A7 centre (261.2, 72.7) radius 9.775
  line L7 (274.2, 3) -> (274.2, 82.7)
  circle A8 centre (261.2, 13) radius 9.775
  dimension "d128" = 19.55
  dimension "d129" = 13
  dimension "d130" = 13
  dimension "d131" = 19.55
  dimension "d132" = 13
  dimension "d133" = 13
  dimension "d134" = 19.55
  dimension "d135" = 13
  dimension "d136" = 13
  dimension "d137" = 19.55
  dimension "d138" = 13
  dimension "d139" = 13
  measures "d128" diameter of A5
  measures "d129" distance of A5.centre L4
  measures "d130" distance of A5.centre L5
  measures "d131" diameter of A6
  measures "d132" distance of A6.centre L6
  measures "d133" distance of L5 A6.centre
  measures "d134" diameter of A7
  measures "d135" distance of L4 A7.centre
  measures "d136" distance of A7.centre L7
  measures "d137" diameter of A8
  measures "d138" distance of L7 A8.centre
  measures "d139" distance of L6 A8.centre
extrude "Extrude14" cut sketch "Sketch16" against normal blind 0.75 contours A5 | A6 | A7 | A8
